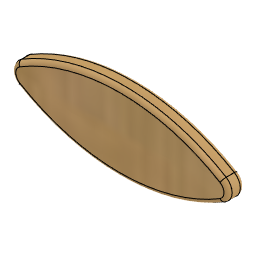
Lamello Size 10 (Autodesk Fusion 360 design; units mm, degrees)
description: Lamello Bisquit
part number: S10
Autodesk Fusion 360 part; units mm, degrees
sketch "Sketch1" plane through (0, 0, 0) normal (0, 0, 1) x (1, 0, 0)
  line L0 (31.5, -2) -> (-31.5, -2)
  line L1 (-31.5, -2) -> (-31.5, 2)
  line L2 (-31.5, 2) -> (31.5, 2)
  line L3 (31.5, 2) -> (31.5, -2)
  line L4 (31.5, -2) -> (-31.5, 2) construction
  line L5 (-31.5, -2) -> (31.5, 2) construction
  dimension "d8" = 4
  dimension "d9" = 63
  constraint horizontal L0
  constraint perpendicular L0 L1
  constraint parallel L0 L2
  constraint parallel L1 L3
  constraint coincident L4 origin
  constraint coincident L5 origin
  measures "d8" distance of L0 L2
  measures "d9" distance of L1 L3
extrude "Extrude1" add sketch "Sketch1" along normal mid plane 20 makes body 1
sketch "Sketch2" plane through (0, 0, 0) normal (0, 1, 0) x (1, 0, 0)
  arc A0 (25.0416, 2.5736) -> (-25.0416, 2.5736) centre (0, -39.2308) ccw
  arc A1 (-25.0416, -2.5736) -> (25.0416, -2.5736) centre (0, 39.2308) ccw
  circle A2 centre (-23.5, 0) radius 3
  circle A3 centre (23.5, 0) radius 3
  point P0 (-26.5, 0)
  point P1 (26.5, 0)
  point P2 (0, 9.5)
  point P3 (0, -9.5)
  dimension "d12" = 6
  dimension "d13" = 6
  dimension "d14" = 53
  dimension "d15" = 19
  constraint vertical origin A1.centre
  constraint vertical origin A0.centre
  constraint vertical A0.end A1.start
  constraint vertical A0.start A1.end
  constraint horizontal origin A2.centre
  constraint coincident A0.end A2
  constraint coincident A1.start A2
  constraint tangent A0 A2
  constraint tangent A1 A2
  constraint horizontal origin A3.centre
  constraint coincident A0.start A3
  constraint tangent A0 A3
  constraint coincident A2 P0
  constraint coincident A3 P1
  constraint horizontal origin P0
  constraint horizontal origin P1
  constraint coincident A1 P3
  constraint vertical origin P2
  constraint vertical origin P3
  constraint coincident A0 P2
  measures "d12" diameter of A2
  measures "d13" diameter of A3
  measures "d14" distance of P0 P1
  measures "d15" distance of P2 P3
extrude "Extrude2" add sketch "Sketch2" along normal mid plane 4 separate body makes body 2
fillet "Fillet1" radius 1 8 edges at (0, 2, -9.5) (-26.5, 2, 0) (0, 2, 9.5) (26.5, 2, 0) (0, -2, -9.5) (26.5, -2, 0) (0, -2, 9.5) (-26.5, -2, 0) on bodies 2
sketch "Sketch4" plane through (0, 0, 0) normal (0, 0, 1) x (1, 0, 0)
hidden bodies 1
equation "LamelloLength = 53 mm" comment "Size20 = 56mm; Size10 = 53 mm; Size0 = 47 mm; SizeH9 = 38 mm"
equation "LamelloWidth = 19 mm" comment "Size20 = 23mm; Size10 = 19mm; Size0 = 15 mm; SizeH9 =12 mm"
equation "LamelloThickness = 4 mm" comment "Size20 = 4mm; Size10 = 4 mm; Size0 = 4 mm; SizeH9 = 3mm"
equation "Tolerance = 1 mm" comment "Recommended tolerance for cutting"
equation "GrooveLength = LamelloLength + Tolerance + 9 mm"
equation "GrooveWidth = LamelloWidth + 1 mm"
equation "GrooveThickness = LamelloThickness"
equation "d8 = GrooveThickness"
equation "d9 = GrooveLength"
equation "d10 = GrooveWidth"
equation "d14 = LamelloLength"
equation "d15 = LamelloWidth"
equation "d16 = LamelloThickness"
named bodies: "Lamello Hole", "Lamello"
